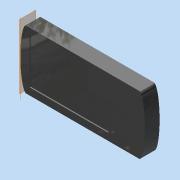
# Autodesk Inventor part: SprintSamsungGalaxyS
Saved by Autodesk Inventor 2011 SP1 (Build 150282100, 282)
## iProperties
Created: 2011-08-14
Part Number: SprintSamsungGalaxyS
Document SubType Name: Modeling
Designer: dgitz
Density: 1 g/cm^3
Author: dgitz
Autodesk Inventor part; units mm, degrees
ref_plane "XZ Plane" through (0, 0, 0) normal (0, 1, 0) x (-1, 0, 0)
ref_plane "XY Plane" through (0, 0, 0) normal (0, 0, 1) x (1, 0, 0)
sketch "Sketch1" plane through (0, 0, 0) normal (0, 0, 1) x (1, 0, 0)
  line L0 (-62.23, 32.385) -> (62.23, 32.385)
  line L1 (62.23, -32.385) -> (-62.23, -32.385)
  line L2 (62.23, 0) -> (68.58, 0) construction
  line L3 (-62.23, 0) -> (-68.58, 0) construction
  ellipse E0 centre (-62.23, 0) end of major axis (-68.58, 0) minor radius 32.385 (-62.23, 32.385) -> (-62.23, -32.385) ccw
  ellipse E1 centre (62.23, 0) end of major axis (68.58, 0) minor radius 32.385 (62.23, -32.385) -> (62.23, 32.385) ccw
  point P0 (0, 0)
  dimension "d2" = 64.77
  dimension "d3" = 32.385
  dimension "d4" = 6.35
  dimension "d5" = 6.35
  dimension "d6" = 62.23
  dimension "d7" = 68.58
  constraints: 8 end point, 7 horizontal, 2 coincident, 2 parallel, 1 collinear, 10 other
  measures "d2" distance between parallel lines of L1 L0
  measures "d3" distance from line of point (0, 0) L0
  measures "d4" distance of L2.start L2.end
  measures "d5" distance of L3.start L3.end
  measures "d6" distance of point (0, 0) point (-62.23, 0)
  measures "d7" distance of L2.end point (0, 0)
extrude "Extrusion1" add sketch "Sketch1" along normal blind 16.256
ref_plane "Work Plane1" through (-68.58, 0, 0) normal (1, 0, 0) x (0, 1, 0)
sketch "Sketch2" plane through (0, 0, 0) normal (1, 0, 0) x (0, 1, 0)
  point P0 (0, 0)
sketch "Sketch3" plane through (-68.58, 0, 0) normal (1, 0, 0) x (0, 1, 0)
  circle A0 centre (-15.5448, 4.1402) radius 1.6002
  line L0 (-32.385, 0) -> (32.385, 0) projected
  line L1 (-32.385, 0) -> (-32.385, 16.256) projected
  point P0 (0, 0)
  dimension "d10" = 3.2004
  dimension "d11" = 2.54
  dimension "d12" = 15.24
  constraints: 1 centre point
  measures "d10" diameter of A0
  measures "d11" distance edge to line of A0 L0
  measures "d12" distance edge to line of A0 L1
extrude "Extrusion2" cut sketch "Sketch3" along normal blind 9.525
sketch "Sketch4" plane through (-68.58, 0, 0) normal (1, 0, 0) x (0, 1, 0)
  line L0 (3.937, 2.794) -> (-6.985, 2.794)
  line L1 (-6.985, 2.794) -> (-6.985, 6.223)
  line L2 (-6.985, 6.223) -> (3.937, 6.223)
  line L3 (3.937, 6.223) -> (3.937, 2.794)
  line L4 (-32.385, 0) -> (32.385, 0) projected
  line L5 (-32.385, 0) -> (-32.385, 16.256) projected
  point P0 (0, 0)
  dimension "d15" = 3.429
  dimension "d16" = 10.922
  dimension "d17" = 2.794
  dimension "d18" = 25.4
  constraints: 8 end point, 2 parallel, 1 horizontal, 1 perpendicular
  measures "d15" distance between parallel lines of L2 L0
  measures "d16" distance between parallel lines of L1 L3
  measures "d17" distance between parallel lines of L0 L4
  measures "d18" distance between parallel lines of L1 L5
extrude "Extrusion3" cut sketch "Sketch4" along normal blind 2.54
sketch "Sketch5" plane through (0, 0, 16.256) normal (0, 0, 1) x (1, 0, 0)
  line L0 (-62.23, 32.385) -> (62.23, 32.385) projected
  line L1 (-58.42, 26.1874) -> (28.448, 26.1874)
  line L2 (28.448, 26.1874) -> (28.448, -24.6126)
  line L3 (28.448, -24.6126) -> (-58.42, -24.6126)
  line L4 (-58.42, -24.6126) -> (-58.42, 26.1874)
  point P0 (0, 0)
  dimension "d21" = 50.8
  dimension "d22" = 86.868
  dimension "d23" = 3.81
  dimension "d24" = 6.1976
  constraints: 8 end point, 2 parallel, 1 horizontal, 1 perpendicular
  measures "d21" distance between parallel lines of L3 L1
  measures "d22" distance between parallel lines of L2 L4
  measures "d23" distance from line of L0.start L4
  measures "d24" distance between parallel lines of L0 L1
extrude "Extrusion4" cut sketch "Sketch5" against normal blind 1.27
body "Solid1"
